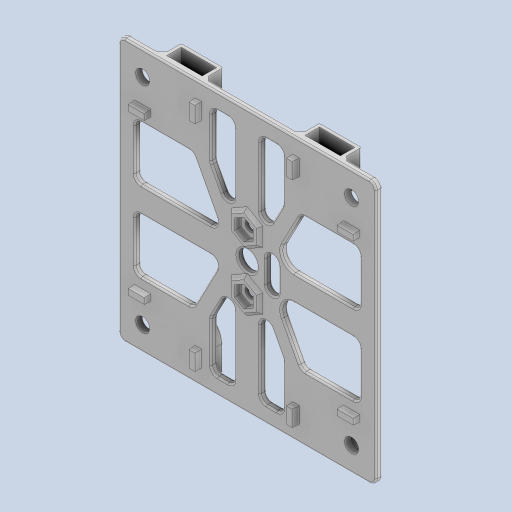
# Autodesk Inventor part: BLTouch-Leveling-Plate_V2
Saved by Autodesk Inventor 2023.2 (Build 272271000, 271)
## iProperties
Created: 2024-02-15
Part Number: BLTouch-Leveling-Plate_V2
Material: Generisch
Document SubType Name: Modeling
Designer: Nils Bade
Density: 1 g/cm^3
Appearance: Vorgabe
Description: Dummy
Auf Bestellliste: True
Author: Nils Bade
Autodesk Inventor part; units mm, degrees
ref_plane "YZ Plane" through (0, 0, 0) normal (1, 0, 0) x (0, 1, 0)
ref_plane "XY Plane" through (0, 0, 0) normal (0, 0, 1) x (1, 0, 0)
sketch "S-Basis" plane through (0, 0, 0) normal (0, 0, 1) x (1, 0, 0)
  line L0 (0, 57.19) -> (0, -57.19) construction
  line L1 (-56, 0) -> (56, 0) construction
  line L2 (-40, 40.85) -> (40, 40.85)
  line L3 (40, 40.85) -> (40, -40.85)
  line L4 (40, -40.85) -> (-40, -40.85)
  line L5 (-40, -40.85) -> (-40, 40.85)
  line L6 (-40, 40.85) -> (40, -40.85) construction
  line L7 (40, 40.85) -> (-40, -40.85) construction
  line L8 (-40, 33.35) -> (40, 33.35) construction
  line L9 (-40, 13.03) -> (40, 13.03) construction
  circle A0 centre (32.5, 33.35) radius 2.15
  circle A1 centre (-32.5, -33.35) radius 2.15
  circle A2 centre (32.5, -33.35) radius 2.15
  line L10 (-40, -40.85) -> (-16.2, -40.85) construction
  line L11 (-16.2, -40.85) -> (-16.2, -25.85) construction
  line L12 (-16.2, -25.85) -> (-40, -25.85) construction
  line L13 (-40, -25.85) -> (-40, -40.85) construction
  line L14 (-40, 40.85) -> (-16.2, 40.85) construction
  line L15 (-16.2, 40.85) -> (-16.2, 25.85) construction
  line L16 (-16.2, 25.85) -> (-40, 25.85) construction
  line L17 (-40, 25.85) -> (-40, 40.85) construction
  line L18 (40, -40.85) -> (16.2, -40.85) construction
  line L19 (16.2, -40.85) -> (16.2, -25.85) construction
  line L20 (16.2, -25.85) -> (40, -25.85) construction
  line L21 (40, -25.85) -> (40, -40.85) construction
  line L22 (40, 40.85) -> (16.2, 40.85) construction
  line L23 (40, 25.85) -> (40, 40.85) construction
  line L24 (16.2, 25.85) -> (40, 25.85) construction
  line L25 (16.2, 40.85) -> (16.2, 25.85) construction
  line L26 (-16.2, -35.85) -> (-14.2, -35.85)
  line L27 (-14.2, -35.85) -> (-14.2, -30.85)
  line L28 (-14.2, -30.85) -> (-16.2, -30.85)
  line L29 (-16.2, -30.85) -> (-16.2, -35.85)
  line L30 (-35, -25.85) -> (-30, -25.85)
  line L31 (-30, -25.85) -> (-30, -23.85)
  line L32 (-30, -23.85) -> (-35, -23.85)
  line L33 (-35, -23.85) -> (-35, -25.85)
  line L34 (-16.2, 35.85) -> (-14.2, 35.85)
  line L35 (-14.2, 35.85) -> (-14.2, 30.85)
  line L36 (-14.2, 30.85) -> (-16.2, 30.85)
  line L37 (-16.2, 30.85) -> (-16.2, 35.85)
  line L38 (-35, 25.85) -> (-30, 25.85)
  line L39 (-30, 25.85) -> (-30, 23.85)
  line L40 (-30, 23.85) -> (-35, 23.85)
  line L41 (-35, 23.85) -> (-35, 25.85)
  line L42 (16.2, -35.85) -> (14.2, -35.85)
  line L43 (14.2, -35.85) -> (14.2, -30.85)
  line L44 (14.2, -30.85) -> (16.2, -30.85)
  line L45 (16.2, -30.85) -> (16.2, -35.85)
  line L46 (35, -25.85) -> (30, -25.85)
  line L47 (30, -25.85) -> (30, -23.85)
  line L48 (30, -23.85) -> (35, -23.85)
  line L49 (35, -23.85) -> (35, -25.85)
  line L50 (14.2, 30.85) -> (16.2, 30.85)
  line L51 (14.2, 35.85) -> (14.2, 30.85)
  line L52 (16.2, 35.85) -> (14.2, 35.85)
  line L53 (16.2, 30.85) -> (16.2, 35.85)
  line L54 (30, 25.85) -> (30, 23.85)
  line L55 (30, 23.85) -> (35, 23.85)
  line L56 (35, 23.85) -> (35, 25.85)
  line L57 (35, 25.85) -> (30, 25.85)
  circle A3 centre (-32.5, 33.35) radius 2.15
  point P0 (-16.2, -33.35)
  point P1 (-16.2, 33.35)
  point P2 (16.2, -33.35)
  point P3 (16.2, 33.35)
  dimension "d0" = 81.7
  dimension "d1" = 80
  dimension "d9" = 4.3
  dimension "d10" = 32.5
  dimension "d11" = 7.5
  dimension "d26" = 15
  dimension "d27" = 23.8
  dimension "d30" = 5
  dimension "d31" = 5
  dimension "d32" = 5
  dimension "d33" = 2
  dimension "d34" = 2
  constraints: 112 end point, 38 symmetric about line, 8 parallel, 6 perpendicular, 6 point on line, 4 centre point, 4 horizontal, 2 midpoint, 2 other
  measures "d0" distance of L2.end L3.end
  measures "d1" distance of L2.start L2.end
  measures "d9" diameter of A1
  measures "d10" distance from line of L0 A1.centre
  measures "d11" distance from line of L4 A1.centre
  measures "d26" distance between parallel lines of L4 L12
  measures "d27" distance between parallel lines of L5 L11
  measures "d30" distance between parallel lines of L28 L26
  measures "d31" distance between parallel lines of L31 L33
  measures "d32" distance between parallel lines of L5 L33
  measures "d33" distance between parallel lines of L12 L32
  measures "d34" distance between parallel lines of L11 L27
ref_plane "Anschlussebene-Übergang" through (-40, 13.03, 0) normal (0, 1, 0) x (1, 0, 0)
extrude "Ex-Base1" add sketch "S-Basis" against normal blind 2 contours L2 L3 L4 L5 | L29 L28 L27 L26 | L33 L32 L31 L30 | L34 L35 L36 L37 | L38 L39 L40 L41 | L42 L43 L44 L45 | L46 L47 L48 L49 | L51 L52 L53 L50 | L57 L56 L55 L54
fillet "Rundung-Base" radius 2 4 edges at (40, -40.85, -1) (-40, -40.85, -1) (40, 40.85, -1) (-40, 40.85, -1)
extrude "Ex-Platte-ProbeHead-Formschluss" add sketch "S-Basis" along normal blind 2 contours L29 L28 L27 L26 | L33 L32 L31 L30
chamfer "Fase-formschluss-1" distance 2 angle 5 1 edges at (-16.2, -33.35, 2) measured on face at (-16.2, -33.35, 1.5)
chamfer "Fase-formschluss-2" distance 2 angle 5 1 edges at (-32.5, -25.85, 2) measured on face at (-32.5, -25.85, 1.5)
mirror "Spiegeln1" about plane through (0, 0, 0) normal (0, 1, 0) of "Ex-Platte-ProbeHead-Formschluss", "Fase-formschluss-1", "Fase-formschluss-2"
mirror "Spiegeln2" about plane through (0, 0, 0) normal (1, 0, 0) of "Ex-Platte-ProbeHead-Formschluss", "Fase-formschluss-1", "Fase-formschluss-2", "Spiegeln1"
sketch "S-ResinSave" plane through (0, 0, 0) normal (0, 0, 1) x (1, 0, 0)
  line L0 (0, 57.19) -> (0, -57.19) construction
  line L1 (-35, -4) -> (-35, -20.85)
  line L2 (-35, -20.85) -> (-16.8473, -20.85)
  line L3 (-16.8473, -20.85) -> (-8, -4)
  line L4 (-8, -4) -> (-35, -4)
  line L5 (-11.2, -20.85) -> (-11.2, -35.85)
  line L6 (-11.2, -35.85) -> (-4, -35.85)
  line L7 (-4, -35.85) -> (-4, -7.1374)
  line L8 (-4, -7.1374) -> (-11.2, -20.85)
  line L9 (-35, -23.85) -> (-35, -25.675) construction
  line L10 (-14.2, -35.85) -> (-14.2, -30.85) construction
  line L11 (-30, -23.85) -> (-35, -23.85) construction
  line L12 (-16.025, -35.85) -> (-14.2, -35.85) construction
  line L13 (-56, 0) -> (56, 0) construction
  line L14 (-30, 23.85) -> (-35, 23.85) construction
  line L15 (35, -4) -> (35, -20.85)
  line L16 (35, -20.85) -> (16.8473, -20.85)
  line L17 (16.8473, -20.85) -> (8, -4)
  line L18 (8, -4) -> (35, -4)
  line L19 (11.2, -20.85) -> (11.2, -35.85)
  line L20 (11.2, -35.85) -> (4, -35.85)
  line L21 (4, -35.85) -> (4, -7.1374)
  line L22 (4, -7.1374) -> (11.2, -20.85)
  line L23 (-35, 4) -> (-35, 20.85)
  line L24 (-35, 20.85) -> (-16.8473, 20.85)
  line L25 (-16.8473, 20.85) -> (-8, 4)
  line L26 (-8, 4) -> (-35, 4)
  line L27 (-11.2, 20.85) -> (-11.2, 35.85)
  line L28 (-11.2, 35.85) -> (-4, 35.85)
  line L29 (-4, 35.85) -> (-4, 7.1374)
  line L30 (-4, 7.1374) -> (-11.2, 20.85)
  line L31 (35, 4) -> (35, 20.85)
  line L32 (8, 4) -> (35, 4)
  line L33 (16.8473, 20.85) -> (8, 4)
  line L34 (35, 20.85) -> (16.8473, 20.85)
  line L35 (11.2, 20.85) -> (11.2, 35.85)
  line L36 (4, 7.1374) -> (11.2, 20.85)
  line L37 (4, 35.85) -> (4, 7.1374)
  line L38 (11.2, 35.85) -> (4, 35.85)
  point P0 (0, 0)
  dimension "d74" = 4
  dimension "d75" = 3
  dimension "d76" = 3
  dimension "d77" = 5
  dimension "d78" = 4
  constraints: 64 end point, 24 symmetric about line, 4 point on line, 2 collinear, 2 parallel, 2 perpendicular, 2 vertical
  measures "d74" distance between parallel lines of L0 L7
  measures "d75" distance between parallel lines of L10 L5
  measures "d76" distance between parallel lines of L11 L2
  measures "d77" distance between parallel lines of L8 L3
  measures "d78" distance between parallel lines of L4 L13
extrude "Ex-ResinSave" cut sketch "S-ResinSave" against normal blind 2
fillet "Run1-ResinSave" radius 2 30 edges at (-4, -7.1374, -1) (-8, -4, -1) (4, -7.1374, -1) (4, 7.1374, -1) (-4, 7.1374, -1) (-8, 4, -1) (11.2, 35.85, -1) (4, 35.85, -1) (11.2, 20.85, -1) (16.8473, 20.85, -1) (35, 20.85, -1) (35, 4, -1) (35, -20.85, -1) (16.8473, -20.85, -1) (35, -4, -1) (11.2, -35.85, -1) (11.2, -20.85, -1) (4, -35.85, -1) (-4, -35.85, -1) (-11.2, -35.85, -1) (-11.2, -20.85, -1) (-16.8473, -20.85, -1) (-35, -4, -1) (-35, -20.85, -1) (-16.8473, 20.85, -1) (-35, 4, -1) (-35, 20.85, -1) (-11.2, 20.85, -1) (-11.2, 35.85, -1) (-4, 35.85, -1)
fillet "Run2-ResinSave" radius 4 2 edges at (8, -4, -1) (8, 4, -1)
sketch "S-BLTouchAnschraubung" plane through (0, 0, 0) normal (0, 0, 1) x (1, 0, 0)
  circle A0 centre (0, 0) radius 3
  line L0 (0, 18.9047) -> (0, -18.9047) construction
  line L1 (-6.63, 0) -> (12.48, 0) construction
  circle A1 centre (0, -9) radius 1.65
  line L2 (2.9, -10.6743) -> (0, -12.3486)
  line L3 (0, -12.3486) -> (-2.9, -10.6743)
  line L4 (-2.9, -10.6743) -> (-2.9, -7.3257)
  line L5 (-2.9, -7.3257) -> (0, -5.6514)
  line L6 (0, -5.6514) -> (2.9, -7.3257)
  line L7 (2.9, -7.3257) -> (2.9, -10.6743)
  line L8 (3.9, -11.2517) -> (0, -13.5033)
  line L9 (0, -13.5033) -> (-3.9, -11.2517)
  line L10 (-3.9, -11.2517) -> (-3.9, -6.7483)
  line L11 (-3.9, -6.7483) -> (0, -4.4967)
  line L12 (0, -4.4967) -> (3.9, -6.7483)
  line L13 (3.9, -6.7483) -> (3.9, -11.2517)
  circle A2 centre (0, 9) radius 1.65
  line L14 (2.9, 10.6743) -> (0, 12.3486)
  line L15 (0, 12.3486) -> (-2.9, 10.6743)
  line L16 (-2.9, 10.6743) -> (-2.9, 7.3257)
  line L17 (-2.9, 7.3257) -> (0, 5.6514)
  line L18 (0, 5.6514) -> (2.9, 7.3257)
  line L19 (2.9, 7.3257) -> (2.9, 10.6743)
  line L20 (3.9, 11.2517) -> (0, 13.5033)
  line L21 (0, 13.5033) -> (-3.9, 11.2517)
  line L22 (-3.9, 11.2517) -> (-3.9, 6.7483)
  line L23 (-3.9, 6.7483) -> (0, 4.4967)
  line L24 (0, 4.4967) -> (3.9, 6.7483)
  line L25 (3.9, 6.7483) -> (3.9, 11.2517)
  line L26 (7.75, 3.5) -> (7.75, -3.5) construction
  line L27 (5.75, 3.5) -> (5.75, -3.5)
  line L28 (9.75, -3.5) -> (9.75, 3.5)
  arc A3 (9.75, 3.5) -> (5.75, 3.5) centre (7.75, 3.5) ccw
  arc A4 (5.75, -3.5) -> (9.75, -3.5) centre (7.75, -3.5) ccw
  point P0 (7.75, 0)
  point P1 (7.75, -5.5)
  point P2 (7.75, 5.5)
  dimension "d85" = 6
  dimension "d86" = 3.3
  dimension "d87" = 9
  dimension "d88" = 5.8
  dimension "d89" = 1
  dimension "d90" = 5.75
  dimension "d91" = 4
  dimension "d92" = 11
  constraints: 56 end point, 13 symmetric about line, 6 point on circle, 5 centre point, 4 tangent, 2 coincident, 2 point on line, 1 midpoint, 1 parallel, 1 perpendicular, 1 vertical, 19 other
  measures "d85" diameter of A0
  measures "d86" diameter of A1
  measures "d87" distance from line of L1 A1.centre
  measures "d88" distance between parallel lines of L5 L2
  measures "d89" distance between parallel lines of L7 L13
  measures "d90" distance between parallel lines of L0 L27
  measures "d91" distance between parallel lines of L28 L27
  measures "d92" distance of point (7.75, -5.5) point (7.75, 5.5)
extrude "Ex-BLTouchAnschraubung1" cut sketch "S-BLTouchAnschraubung" against normal blind 2 contours A0 | A1 | A2 | A3 L28 A4 L27
extrude "Ex-BLTouchAnschraubung2" cut sketch "S-BLTouchAnschraubung" against normal blind 1 contours L2 L3 L4 L5 L6 L7 | L19 L18 L17 L16 L15 L14
extrude "Ex-BLTouchAnschraubung3" add sketch "S-BLTouchAnschraubung" along normal blind 1 contours L8 L9 L10 L11 L12 L13 | L25 L24 L23 L22 L21 L20
sketch "S-Magnetslots" plane through (0, 0, -2) normal (0, 0, -1) x (-1, 0, 0)
  circle A0 centre (32.5, -33.35) radius 2.15 projected
  line L0 (-38, -40.85) -> (38, -40.85) projected
  line L1 (40, -38.85) -> (40, 38.85) projected
  circle A1 centre (21.5, -33.35) radius 5.5
  line L2 (32.5, -33.35) -> (12.3218, -33.35) construction
  circle A2 centre (21.5, -33.35) radius 6.5
  line L3 (28, -33.35) -> (28, -40.85)
  line L4 (38, -40.85) -> (-38, -40.85) construction
  line L5 (27, -33.35) -> (27, -40.85)
  line L6 (16, -33.35) -> (16, -40.85)
  line L7 (15, -33.35) -> (15, -40.85)
  point P0 (0, 0)
  dimension "d100" = 11
  dimension "d101" = 11
  dimension "d102" = 1
  constraints: 10 end point, 8 point on line, 2 perpendicular, 2 point on circle, 1 centre point, 1 horizontal, 1 parallel, 1 tangent, 1 vertical, 3 other
  measures "d101" distance of L2.start A2.centre
extrude "Ex-Magnetslots1" add sketch "S-Magnetslots" along normal blind 4.5 contours L7 A2 L6 L0 | A2 L5 A1 L6 | L5 A2 L3 L0 picked at (15.817, -35.2977)
extrude "Ex-Magnetslots2" add sketch "S-Magnetslots" along normal blind 1 from surface at 4.5 contours L7 A2 L6 L0 | L6 A2 L5 L0 | A2 L5 A1 L6 | L5 A2 L3 L0 | L6 A1 L5 A2 | A1
mirror "Spiegeln3" about plane through (0, 0, 0) normal (0, 1, 0) of "Ex-Magnetslots1", "Ex-Magnetslots2"
mirror "Spiegeln4" about plane through (0, 0, 0) normal (1, 0, 0) of "Ex-Magnetslots1", "Ex-Magnetslots2", "Spiegeln3"
chamfer "Fase-1mm" distance 1 angle 45 24 edges at (-15, -37.1, -2) (-21.5, -26.85, -2) (-28, -37.1, -2) (21.5, -26.85, -2) (15, -37.1, -2) (28, -37.1, -2) (15, 37.1, -2) (21.5, 26.85, -2) (28, 37.1, -2) (-21.5, 26.85, -2) (-15, 37.1, -2) (-28, 37.1, -2) (-3.9, -9, 0) (-1.95, -12.3775, 0) (1.95, -12.3775, 0) (3.9, -9, 0) (-1.95, -5.6225, 0) (1.95, -5.6225, 0) (1.95, 5.6225, 0) (-1.95, 5.6225, 0) (3.9, 9, 0) (1.95, 12.3775, 0) (-1.95, 12.3775, 0) (-3.9, 9, 0)
fillet "Rundung-0.5mm" radius 0.5 170 edges at (7.75, 5.5, -2) (5.75, 0, -2) (7.75, -5.5, -2) (9.75, 0, -2) (7.75, -5.5, 0) (5.75, 0, 0) (7.75, 5.5, 0) (9.75, 0, 0) (-3, 0, 0) (-3, 0, -2) (34.4142, -4.5858, 0) (35, -12.425, 0) (34.4142, -20.2642, 0) (25.5281, -20.85, 0) (17.0216, -20.5617, 0) (13.681, -14.8196, 0) (11.1948, -5.9309, 0) (23.8091, -4, 0) (11.1948, -5.9309, -2) (13.681, -14.8196, -2) (17.0216, -20.5617, -2) (25.5281, -20.85, -2) (34.4142, -20.2642, -2) (35, -12.425, -2) (34.4142, -4.5858, -2) (23.8091, -4, -2) (34.4142, 4.5858, 0) (23.8091, 4, 0) (11.1948, 5.9309, 0) (13.681, 14.8196, 0) (17.0216, 20.5617, 0) (25.5281, 20.85, 0) (34.4142, 20.2642, 0) (35, 12.425, 0) (34.4142, 20.2642, -2) (25.5281, 20.85, -2) (17.0216, 20.5617, -2) (13.681, 14.8196, -2) (11.1948, 5.9309, -2) (23.8091, 4, -2) (34.4142, 4.5858, -2) (35, 12.425, -2) (11.1418, 20.8643, 0) (9.3707, 17.3661, 0) (5.5212, 13.3068, 0) (4, 24.5493, 0) (4.5858, 35.2642, 0) (7.6, 35.85, 0) (10.6142, 35.2642, 0) (11.2, 27.5966, 0) (10.6142, 35.2642, -2) (7.6, 35.85, -2) (4.5858, 35.2642, -2) (4, 24.5493, -2) (5.5212, 13.3068, -2) (9.3707, 17.3661, -2) (11.1418, 20.8643, -2) (11.2, 27.5966, -2) (-5.5212, 13.3068, 0) (-9.3707, 17.3661, 0) (-11.1418, 20.8643, 0) (-11.2, 27.5966, 0) (-10.6142, 35.2642, 0) (-7.6, 35.85, 0) (-4.5858, 35.2642, 0) (-4, 24.5493, 0) (-4.5858, 35.2642, -2) (-7.6, 35.85, -2) (-10.6142, 35.2642, -2) (-11.2, 27.5966, -2) (-11.1418, 20.8643, -2) (-9.3707, 17.3661, -2) (-5.5212, 13.3068, -2) (-4, 24.5493, -2) (-9.5974, 4.9655, 0) (-22.1545, 4, 0) (-34.4142, 4.5858, 0) (-35, 12.425, 0) (-34.4142, 20.2642, 0) (-25.5281, 20.85, 0) (-17.0216, 20.5617, 0) (-12.9118, 13.3548, 0) (-17.0216, 20.5617, -2) (-25.5281, 20.85, -2) (-34.4142, 20.2642, -2) (-35, 12.425, -2) (-34.4142, 4.5858, -2) (-22.1545, 4, -2) (-9.5974, 4.9655, -2) (-12.9118, 13.3548, -2) (-17.0216, -20.5617, 0) (-25.5281, -20.85, 0) (-34.4142, -20.2642, 0) (-35, -12.425, 0) (-34.4142, -4.5858, 0) (-22.1545, -4, 0) (-9.5974, -4.9655, 0) (-12.9118, -13.3548, 0) (-9.5974, -4.9655, -2) (-22.1545, -4, -2) (-34.4142, -4.5858, -2) (-35, -12.425, -2) (-34.4142, -20.2642, -2) (-25.5281, -20.85, -2) (-17.0216, -20.5617, -2) (-12.9118, -13.3548, -2) (-4.5858, -35.2642, 0) (-7.6, -35.85, 0) (-10.6142, -35.2642, 0) (-11.2, -27.5966, 0) (-11.1418, -20.8643, 0) (-9.3707, -17.3661, 0) (-5.5212, -13.3068, 0) (-4, -24.5493, 0) (10.6142, -35.2642, 0) (7.6, -35.85, 0) (4.5858, -35.2642, 0) (4, -24.5493, 0) (5.5212, -13.3068, 0) (9.3707, -17.3661, 0) (11.1418, -20.8643, 0) (11.2, -27.5966, 0) (11.1418, -20.8643, -2) (9.3707, -17.3661, -2) (5.5212, -13.3068, -2) (4, -24.5493, -2) (4.5858, -35.2642, -2) (7.6, -35.85, -2) (10.6142, -35.2642, -2) (11.2, -27.5966, -2) (-5.5212, -13.3068, -2) (-9.3707, -17.3661, -2) (-11.1418, -20.8643, -2) (-11.2, -27.5966, -2) (-10.6142, -35.2642, -2) (-7.6, -35.85, -2) (-4.5858, -35.2642, -2) (-4, -24.5493, -2) (39.4142, -40.2642, 0) (40, 0, 0) (39.4142, 40.2642, 0) (0, 40.85, 0) (-39.4142, 40.2642, 0) (-40, 0, 0) (-39.4142, -40.2642, 0) (0, -40.85, 0) (0, 40.85, -2) (-39.4142, 40.2642, -2) (-40, 0, -2) (-39.4142, -40.2642, -2) (-33.4999, -40.85, -2) (-33.4999, 40.85, -2) (0, -40.85, -2) (40, 0, -2) (39.4142, 40.2642, -2) (33.4999, 40.85, -2) (33.4999, -40.85, -2) (39.4142, -40.2642, -2) (21.5, 26.85, -7.5) (28, 37.1, -7.5) (15, 37.1, -7.5) (-21.5, 26.85, -7.5) (-28, 37.1, -7.5) (-15, 37.1, -7.5) (-28, -37.1, -7.5) (-15, -37.1, -7.5) (-21.5, -26.85, -7.5) (28, -37.1, -7.5) (15, -37.1, -7.5) (21.5, -26.85, -7.5)
equation "\"d10\" = d8"
equation "\"d11\" = d4"
equation "\"d8\" = 32.5"
equation "\"d4\" = 7.5"
